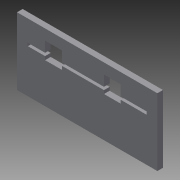
# Autodesk Inventor part: FrontBulkhead
Saved by Autodesk Inventor 2014 (Build 180170000, 170)
## iProperties
Created: 2015-01-07
Part Number: FrontBulkhead
Material: Generic
Document SubType Name: Modeling
Designer: Owner
Density: 1 g/cm^3
Appearance: Default
Author: Owner
Autodesk Inventor part; units mm, degrees
ref_plane "YZ Plane" through (0, 0, 0) normal (1, 0, 0) x (0, 1, 0)
ref_plane "XZ Plane" through (0, 0, 0) normal (0, 1, 0) x (-1, 0, 0)
ref_plane "XY Plane" through (0, 0, 0) normal (0, 0, 1) x (1, 0, 0)
sketch "Sketch1" plane through (0, 0, 0) normal (0, 0, 1) x (1, 0, 0)
  line L0 (60.3753, 90.1264) -> (-18.9997, 90.1264)
  line L1 (-18.9997, 90.1264) -> (-18.9997, 52.0264)
  line L2 (-18.9997, 52.0264) -> (60.3753, 52.0264)
  line L3 (60.3753, 52.0264) -> (60.3753, 90.1264)
  line L4 (60.3753, 78.1884) -> (-18.9997, 78.1884)
  line L5 (-18.9997, 78.1884) -> (-18.9997, 76.5584)
  line L6 (-18.9997, 76.5584) -> (60.3753, 76.5584)
  line L7 (60.3753, 76.5584) -> (60.3753, 78.1884)
  line L8 (54.4063, 78.1884) -> (54.4063, 76.5584)
  line L9 (-12.9037, 76.5584) -> (-12.9037, 78.1884)
  point P0 (0, 0)
  dimension "d0" = 38.1
  dimension "d1" = 79.375
  dimension "d2" = 1.63
  dimension "d3" = 11.938
  dimension "d6" = 67.31
  dimension "d7" = 6.096
  constraints: 20 end point, 6 point on line, 4 parallel, 4 perpendicular, 2 horizontal
  measures "d0" distance of L0.end L1.end
  measures "d1" distance of L0.start L0.end
  measures "d2" distance between parallel lines of L6 L4
  measures "d3" distance between parallel lines of L0 L4
  measures "d6" distance between parallel lines of L8 L9
  measures "d7" distance between parallel lines of L1 L9
extrude "Extrusion1" add sketch "Sketch1" along normal blind 3.175 contours L3 L4 L1 L0 | L3 L6 L8 L4 | L4 L9 L6 L1 | L3 L2 L1 L6
sketch "Sketch2" plane through (0, 0, 0) normal (0, 0, -1) x (-1, 0, 0)
  line L0 (-54.4063, 78.1884) -> (12.9037, 78.1884) projected
  line L1 (-6.3913, 84.1043) -> (3.1337, 84.1043)
  line L2 (3.1337, 84.1043) -> (3.1337, 74.5793)
  line L3 (3.1337, 74.5793) -> (-6.3913, 74.5793)
  line L4 (-6.3913, 74.5793) -> (-6.3913, 84.1043)
  line L5 (-39.708, 84.1761) -> (-30.183, 84.1761)
  line L6 (-30.183, 84.1761) -> (-30.183, 74.6584)
  line L7 (-30.183, 74.6584) -> (-39.708, 74.6584)
  line L8 (-39.708, 74.6584) -> (-39.708, 84.1761)
  line L9 (18.9997, 52.0264) -> (-60.3753, 52.0264) projected
  line L10 (-50.8503, 52.0264) -> (-12.7503, 52.0264)
  line L11 (-60.3753, 90.1264) -> (18.9997, 90.1264) projected
  line L12 (-28.6253, 90.1264) -> (-15.9253, 90.1264)
  point P0 (0, 0)
  dimension "d8" = 9.525
  dimension "d9" = 9.5177
  dimension "d10" = 9.525
  dimension "d11" = 9.525
  dimension "d13" = 5.9159
  constraints: 20 end point, 4 horizontal, 4 parallel, 2 perpendicular, 2 point on line
  measures "d8" distance of L5.start L5.end
  measures "d9" distance of L5.end L6.end
  measures "d10" distance of L1.start L1.end
  measures "d11" distance of L3.end L1.start
  measures "d13" distance between parallel lines of L0 L1
extrude "Extrusion2" cut sketch "Sketch2" against normal blind 3.175
body "Solid1"
